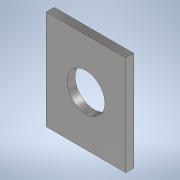
# Autodesk Inventor part: Frame top
Saved by Autodesk Inventor 2020 (Build 240168000, 168)
## iProperties
Created: 2022-06-23
Part Number: Frame top
Material: Steel, Alloy
Document SubType Name: Modeling
Designer: karimi2
Density: 7.73 g/cm^3
Appearance: Semi-Polished
Author: karimi2
Autodesk Inventor part; units mm, degrees
ref_plane "YZ Plane" through (0, 0, 0) normal (1, 0, 0) x (0, 1, 0)
ref_plane "XZ Plane" through (0, 0, 0) normal (0, 1, 0) x (-1, 0, 0)
ref_plane "XY Plane" through (0, 0, 0) normal (0, 0, 1) x (1, 0, 0)
sketch "Sketch1" plane through (0, 0, 0) normal (0, 0, 1) x (1, 0, 0)
  line L0 (0, 0) -> (0, 60) construction
  line L1 (0, 50) -> (-20, 50)
  line L2 (-20, 50) -> (-20, 0)
  line L3 (-20, 0) -> (0, 0)
  line L4 (0, 50) -> (20, 50)
  line L5 (20, 50) -> (20, 0)
  line L6 (20, 0) -> (0, 0)
  circle A0 centre (0, 25) radius 9.5
  dimension "d0" = 60
  dimension "d1" = 50
  dimension "d2" = 20
  dimension "d3" = 19
  constraints: 14 end point, 2 point on line, 2 symmetric about line, 2 vertical, 1 centre point, 1 horizontal, 1 perpendicular
  measures "d0" distance of L0.start L0.end
  measures "d1" distance of L0.start L1.start
  measures "d2" distance of L1.start L1.end
  measures "d3" diameter of A0
extrude "Extrusion1" add sketch "Sketch1" along normal mid plane 4
body "Solid1"
